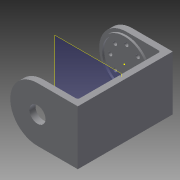
# Autodesk Inventor part: Turnmount
Saved by Autodesk Inventor 2015 (Build 190159000, 159)
## iProperties
Created: 2016-12-14
Part Number: Turnmount
Material: Generic
Document SubType Name: Modeling
Designer: Rudge-Top
Density: 1 g/cm^3
Appearance: Default
Author: Rudge-Top
Autodesk Inventor part; units mm, degrees
ref_plane "YZ Plane" through (0, 0, 0) normal (1, 0, 0) x (0, 1, 0)
ref_plane "XZ Plane" through (0, 0, 0) normal (0, 1, 0) x (-1, 0, 0)
ref_plane "XY Plane" through (0, 0, 0) normal (0, 0, 1) x (1, 0, 0)
sketch "Sketch1" plane through (0, 0, 0) normal (0, 1, 0) x (-1, 0, 0)
  circle A0 centre (0, 0) radius 11.05
  circle A1 centre (0, 0) radius 12.05
  dimension "d0" = 22.1
  dimension "d1" = 24.1
  constraints: 2 centre point, 2 coincident
  measures "d0" diameter of A0
  measures "d1" diameter of A1
extrude "Extrusion1" add sketch "Sketch1" along normal blind 1
sketch "Sketch2" plane through (0, 1, 0) normal (0, 1, 0) x (1, 0, 0)
  arc A0 (0, 13.5) -> (0, -13.5) centre (0, 0) ccw
  line L0 (0, -13.5) -> (17, -13.5)
  line L1 (0, 13.5) -> (17, 13.5) construction
  line L2 (17, -13.5) -> (17, 13.5)
  line L3 (17, -13.5) -> (20, -13.5)
  line L4 (20, -13.5) -> (20, 13.5)
  line L5 (20, 13.5) -> (17, 13.5)
  line L6 (17, 13.5) -> (0, 13.5)
  dimension "d4" = 27
  dimension "d6" = 3
  dimension "d32" = 17
  constraints: 14 end point, 3 horizontal, 2 perpendicular, 2 point on circle, 1 centre point, 1 coincident, 1 collinear, 1 tangent, 1 vertical
  measures "d4" diameter of A0
  measures "d6" distance of L0.end L3.end
  measures "d32" distance of L0.start L0.end
extrude "Extrusion2" add sketch "Sketch2" along normal blind 3
sketch "Sketch3" plane through (0, 1, 0) normal (0, -1, 0) x (1, 0, 0)
  circle A0 centre (0, 0) radius 8
  point P0 (0, 0)
  point P1 (-8, 0)
  point P2 (-5.6569, -5.6569)
  point P3 (0, -8)
  point P4 (5.6569, -5.6569)
  point P5 (8, 0)
  point P6 (5.6569, 5.6569)
  point P7 (0, 8)
  point P8 (-5.6569, 5.6569)
  dimension "d9" = 16
  dimension "d12" = 360
  constraints: 1 coincident, 1 horizontal alignment, 11 other
hole "Hole1" at (-8, 1, 0) at (-5.6569, 1, -5.6569) at (0, 1, -8) at (5.6569, 1, -5.6569) at (8, 1, 0) at (5.6569, 1, 5.6569) at (0, 1, 8) at (-5.6569, 1, 5.6569) direction (0, 1, 0) diameter 2 end through all
sketch "Sketch4" plane through (0, 0, 0) normal (0, -1, 0) x (1, 0, 0)
  point P0 (0, 0)
sketch "Sketch5" plane through (0, 1, 0) normal (0, -1, 0) x (1, 0, 0)
  line L0 (0, 13.5) -> (20, 13.5) projected
  arc A0 (0, 13.5) -> (0, -13.5) centre (0, 0) ccw projected
  line L1 (20, -13.5) -> (0, -13.5) projected
  line L2 (20, 13.5) -> (20, -13.5) projected
  circle A1 centre (0, 0) radius 12.05 projected
  line L3 (20, -13.5) -> (17, -13.5)
  line L4 (17, -13.5) -> (17, 13.5)
  line L5 (17, 13.5) -> (20, 13.5)
  line L6 (20, 13.5) -> (20, -13.5)
  point P0 (0, 0)
  dimension "d21" = 3
  constraints: 8 end point, 2 parallel, 1 horizontal, 1 perpendicular, 1 point on line
  measures "d21" distance of L4.end L5.end
extrude "Extrusion3" add sketch "Sketch5" along normal blind 44.1 contours L0 L2 L1 L4
sketch "Sketch6" plane through (17, 1, -13.5) normal (-1, 0, 0) x (0, 0, 1)
  point P0 (13.5, -1)
ref_plane "Work Plane1" through (0, -19.55, 0) normal (0, 1, 0) x (1, 0, 0)
mirror "Mirror1" about plane through (0, -19.55, 0) normal (0, 1, 0) of "Extrusion2"
sketch "Sketch7" plane through (0, -43.1, 0) normal (0, -1, 0) x (1, 0, 0)
  point P0 (0, 0)
  point P1 (0, 0)
  constraints: 1 coincident
hole "Hole2" at (0, -43.1, 0) direction (0, 1, 0) diameter 8 depth 3 tip angle 118
fillet "Fillet1" radius 1 2 edges at (17, 1, 0) (17, -40.1, 0)
sketch "Sketch8" plane through (20, 4, -13.5) normal (0, 0, -1) x (-1, 0, 0)
  point P0 (20, -4)
body "Solid1"
